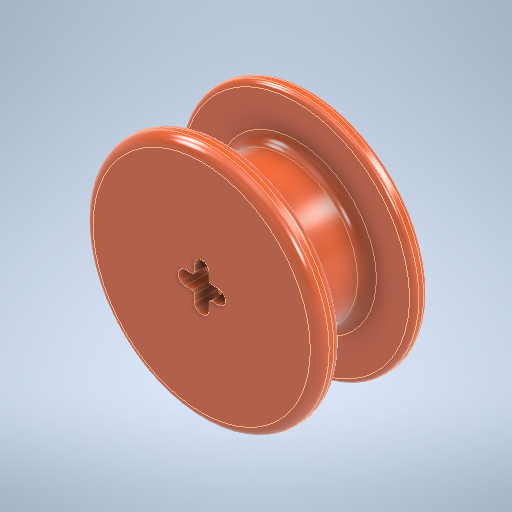
# Autodesk Inventor part: Steering Gear Plate
Saved by Autodesk Inventor 2025.2 (Build 292293000, 293)
## iProperties
Created: 2025-02-06
Part Number: Steering Gear Plate
Material: Generic
Document SubType Name: Modeling
Designer: eason
Density: 1 g/cm^3
Appearance: Smooth - Light Orange
Author: eason
Autodesk Inventor part; units mm, degrees
ref_plane "XZ Plane" through (0, 0, 0) normal (0, 1, 0) x (-1, 0, 0)
sketch "Sketch1" plane through (0, 0, 0) normal (0, 0, 1) x (1, 0, 0)
  circle A0 centre (0, 0) radius 25
  circle A1 centre (0, 0) radius 2
  circle A2 centre (0, 0) radius 5
  circle A3 centre (3.5, 0) radius 1.5
  circle A4 centre (-3.5, 0) radius 1.5
  line L0 (-35, 0) -> (35, 0) projected
  circle A5 centre (0, 3.5) radius 1.5
  circle A6 centre (0, -3.5) radius 1.5
  line L1 (0, -35) -> (0, 35) projected
  line L2 (-1.5, -3.5) -> (-1.5, -2)
  line L3 (-3.5, -1.5) -> (-2, -1.5)
  arc A7 (-1.5, -2) -> (-2, -1.5) centre (-2, -2) ccw
  line L4 (1.5, -3.5) -> (1.5, -2)
  arc A8 (2, -1.5) -> (1.5, -2) centre (2, -2) ccw
  line L5 (3.5, -1.5) -> (2, -1.5)
  line L6 (3.5, 1.5) -> (2, 1.5)
  arc A9 (1.5, 2) -> (2, 1.5) centre (2, 2) ccw
  line L7 (1.5, 3.5) -> (1.5, 2)
  line L8 (-1.5, 3.5) -> (-1.5, 2)
  arc A10 (-2, 1.5) -> (-1.5, 2) centre (-2, 2) ccw
  line L9 (-3.5, 1.5) -> (-2, 1.5)
  point P0 (-5, 0)
  point P1 (-2, 0)
  point P2 (2, 0)
  point P3 (5, 0)
  point P4 (0, -5)
  point P5 (0, -2)
  point P6 (0, 2)
  point P7 (0, 5)
  point P8 (1.5, 3.5)
  point P9 (1.5, -3.5)
  dimension "d0" = 50
  dimension "d2" = 10
  dimension "d60" = 3
  dimension "d61" = 0.5
  dimension "d64" = 360
  constraints: 16 end point, 9 centre point, 8 point on circle, 6 tangent, 4 point on line, 3 coincident, 2 horizontal, 2 vertical, 43 other
  measures "d0" diameter of A0
  measures "d2" diameter of A2
  measures "d60" radial gap between concentric circles of A2 A1
  measures "d61" radius of A7
extrude "Extrusion1" add sketch "Sketch1" along normal blind 5 contours L0 A2 L1 A0 | A0 L1 A2 L0 | L1 A2 L0 A0 | A0 L0 A2 L1 | A3 L6 A9 L7 A5 A2 | A2 A6 L4 A8 L5 A3 | A5 L8 A10 L9 A4 A2 | A2 A4 L3 A7 L2 A6
ref_plane "Work Plane1" through (0, 0, 2.5) normal (0, 0, 1) x (1, 0, 0)
sketch "Sketch9" plane through (0, 0, 0) normal (0, 0, -1) x (-1, 0, 0)
  circle A0 centre (0, 0) radius 15
  circle A1 centre (0, 0) radius 10
  dimension "d75" = 30
  dimension "d76" = 5
  constraints: 2 centre point, 2 coincident
  measures "d75" diameter of A0
  measures "d76" radial gap between concentric circles of A1 A0
extrude "Extrusion9" add sketch "Sketch9" along normal blind 15
sketch "Sketch10" plane through (0, 0, -15) normal (0, 0, -1) x (-1, 0, 0)
  circle A0 centre (0, 0) radius 10 projected
  circle A1 centre (0, 0) radius 25 projected
extrude "Extrusion10" add sketch "Sketch10" along normal blind 3
ref_plane "Work Plane2" through (-15, 0, 0) normal (1, 0, 0) x (0, 1, 0)
sketch "Sketch11" plane through (-15, 0, 0) normal (1, 0, 0) x (0, 1, 0)
  circle A0 centre (0, -7.5) radius 1.5
  line L0 (0, -19) -> (0, 9) projected
  line L1 (25, 0) -> (-25, 0) projected
  point P0 (0, 0)
  dimension "d81" = 3
  dimension "d82" = 7.5
  constraints: 1 centre point, 1 point on line
  measures "d81" diameter of A0
  measures "d82" distance from line of L1 A0.centre
extrude "Extrusion11" cut sketch "Sketch11" along normal up to surface
fillet "Fillet8" radius 2 6 edges at (-25, 0, 5) (-25, 0, 0) (10, 0, 0) (15, 0, 0) (15, 0, -15) (10, 0, -18)
fillet "Fillet9" radius 1 2 edges at (25, 0, -18) (25, 0, -15)
fillet "Fillet10" radius 1 6 edges at (-9.936, 1.1292, -8.4874) (-9.8869, -1.5, -7.5025) (-9.9364, 1.1265, -6.5095) (-14.9248, -1.5, -7.5002) (-14.9576, 1.1271, -6.5102) (-14.9574, 1.1297, -8.4868)
body "Solid1"
